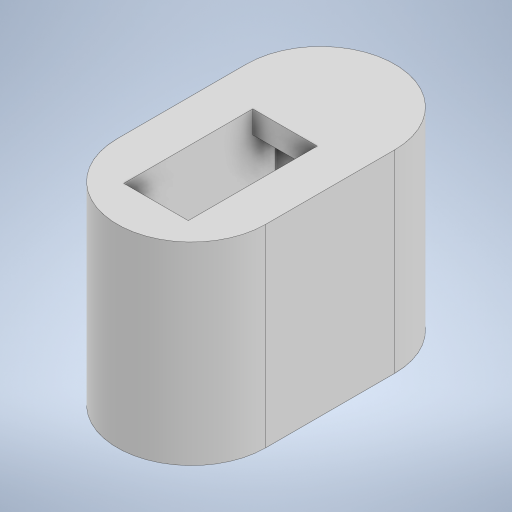
# Autodesk Inventor part: wirst2
Saved by Autodesk Inventor 2023 (Build 270158000, 158)
## iProperties
Created: 2024-06-26
Part Number: wirst2
Material: Generic
Document SubType Name: Modeling
Designer: Swoby
Density: 1 g/cm^3
Appearance: Default
Author: Swoby
Autodesk Inventor part; units mm, degrees
ref_plane "YZ Plane" through (0, 0, 0) normal (1, 0, 0) x (0, 1, 0)
ref_plane "XZ Plane" through (0, 0, 0) normal (0, 1, 0) x (-1, 0, 0)
ref_plane "XY Plane" through (0, 0, 0) normal (0, 0, 1) x (1, 0, 0)
sketch "Sketch1" plane through (0, 0, 0) normal (0, 1, 0) x (-1, 0, 0)
  arc A0 (23, 0) -> (-23, 0) centre (0, 0) ccw
  line L0 (10, 18) -> (-10, 18)
  line L1 (-10, 18) -> (-10, -36)
  line L2 (-10, -36) -> (10, -36)
  line L3 (10, -36) -> (10, 18)
  arc A1 (-23, -40) -> (23, -40) centre (0, -40) ccw
  line L4 (0, 0) -> (0, -40) construction
  line L5 (23, 0) -> (23, -40)
  line L6 (-23, 0) -> (-23, -40)
  arc A2 (10, -20.7123) -> (23, 0) centre (0, 0) ccw construction
  arc A3 (-23, 0) -> (10, -20.7123) centre (0, 0) ccw construction
  arc A4 (-10, -19.2877) -> (-23, -40) centre (0, -40) ccw construction
  arc A5 (23, -40) -> (-10, -19.2877) centre (0, -40) ccw construction
  line L7 (-10, 11) -> (10, 11)
  line L8 (-10, -29) -> (10, -29)
  dimension "d0" = 46
  dimension "d1" = 20
  dimension "d2" = 10
  dimension "d3" = 46
  dimension "d4" = 40
  dimension "d5" = 36
  dimension "d6" = 54
  dimension "d9" = 7
  dimension "d10" = 7
  constraints: 18 end point, 12 point on circle, 8 tangent, 6 centre point, 6 point on line, 2 horizontal, 2 parallel, 2 perpendicular, 1 coincident, 1 vertical
  measures "d0" diameter of A0
  measures "d1" distance of L0.start L0.end
  measures "d2" distance from line of L3 point (0, 0)
  measures "d3" diameter of A1
  measures "d4" distance of L4.end point (0, 0)
  measures "d5" distance from line of L2 point (0, 0)
  measures "d6" distance of L2.end L0.start
  measures "d9" distance between parallel lines of L0 L7
  measures "d10" distance between parallel lines of L2 L8
extrude "Extrusion1" add sketch "Sketch1" along normal blind 60 contours L5 A1 L6 A0 | L3 L7 L1 L0 | L3 L8 L1 L7 | L3 L2 L1 L8
extrude "Extrusion2" cut sketch "Sketch1" along normal through all contours L3 L8 L1 L7
extrude "Extrusion3" cut sketch "Sketch1" along normal blind 53 contours L3 L7 L1 L0 | L3 L2 L1 L8
body "Solid1"
